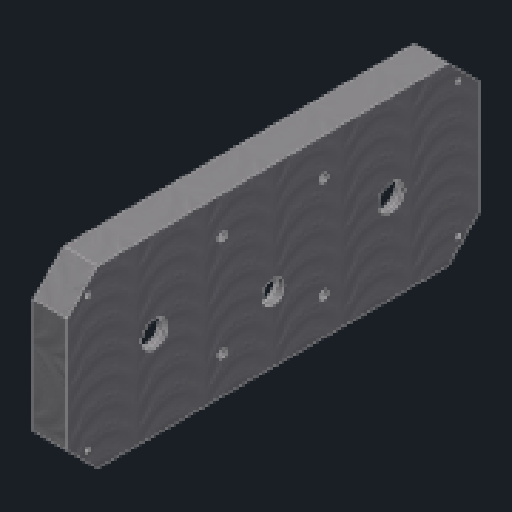
# Autodesk Inventor part: CAJA
Saved by Autodesk Inventor 2024.3 (Build 283343000, 343)
## iProperties
Created: 2024-06-29
Part Number: CAJA
Material: Steel, Mild, Welded
Document SubType Name: Modeling
Designer: Niler
Density: 7.85 g/cm^3
Appearance: Weld - Steel Mild
Author: Niler
Autodesk Inventor part; units mm, degrees
ref_plane "YZ Plane" through (0, 0, 0) normal (1, 0, 0) x (0, 1, 0)
ref_plane "XZ Plane" through (0, 0, 0) normal (0, 1, 0) x (-1, 0, 0)
ref_plane "XY Plane" through (0, 0, 0) normal (0, 0, 1) x (1, 0, 0)
sketch "Sketch1" plane through (0, 0, 0) normal (1, 0, 0) x (0, 1, 0)
  line L0 (-57.5, 135) -> (57.5, 135)
  line L1 (57.5, 135) -> (57.5, -135)
  line L2 (57.5, -135) -> (-57.5, -135)
  line L3 (-57.5, -135) -> (-57.5, 135)
  line L4 (-57.5, 135) -> (57.5, -135) construction
  line L5 (57.5, 135) -> (-57.5, -135) construction
  circle A0 centre (0, 77.5) radius 3.925
  circle A1 centre (0, -77.5) radius 3.925
  circle A2 centre (-15, 0) radius 5
  line L6 (0, 77.5) -> (0, -77.5) construction
  line L7 (51.5, -129) -> (51.5, 129)
  line L8 (51.5, 129) -> (-51.5, 129)
  line L9 (-51.5, 129) -> (-51.5, -129)
  line L10 (-51.5, -129) -> (51.5, -129)
  point P0 (0, 0)
  dimension "d0" = 155
  dimension "d1" = 7.85
  dimension "d2" = 270
  dimension "d3" = 115
  dimension "d4" = 6
  dimension "d35" = 10
  dimension "d36" = 15
  constraints: 22 end point, 4 parallel, 3 centre point, 3 midpoint, 2 perpendicular, 1 equal radius, 1 horizontal, 1 horizontal alignment, 1 vertical, 1 vertical alignment, 3 other
  measures "d0" distance of L6.end L6.start
  measures "d1" diameter of A0
  measures "d2" distance between parallel lines of L2 L0
  measures "d3" distance of L0.start L0.end
  measures "d4" distance between parallel lines of L1 L7
  measures "d35" diameter of A2
  measures "d36" distance of A2.centre point (0, 0)
extrude "Extrusion1" add sketch "Sketch1" along normal blind 8 contours L0 L1 L2 L3 | A0 | A1 | L10 L9 L8 L7
extrude "Extrusion2" add sketch "Sketch1" against normal blind 14.4 contours L0 L1 L2 L3
sketch "Sketch2" plane through (8, 0, 0) normal (1, 0, 0) x (0, 0, -1)
  line L0 (135, -57.5) -> (135, 57.5) projected
  line L1 (135, 57.5) -> (-135, 57.5) projected
  line L2 (-135, 57.5) -> (-135, -57.5) projected
  line L3 (-135, -57.5) -> (135, -57.5) projected
  line L4 (-33.234, -33.234) -> (33.234, -33.234) construction
  line L5 (33.234, -33.234) -> (33.234, 33.234) construction
  line L6 (33.234, 33.234) -> (-33.234, 33.234) construction
  line L7 (-33.234, 33.234) -> (-33.234, -33.234) construction
  line L8 (-33.234, -33.234) -> (33.234, 33.234) construction
  line L9 (33.234, -33.234) -> (-33.234, 33.234) construction
  circle A0 centre (0, 0) radius 47 construction
  circle A1 centre (33.234, 33.234) radius 2.75
  circle A2 centre (-33.234, 33.234) radius 2.75
  circle A3 centre (0, 0) radius 47 construction
  circle A4 centre (-33.234, -33.234) radius 2.75
  circle A5 centre (0, 0) radius 47 construction
  circle A6 centre (33.234, -33.234) radius 2.75
  circle A7 centre (0, 0) radius 47 construction
  point P0 (0, 0)
  point P1 (0, 0)
  dimension "d12" = 94
  dimension "d13" = 5.5
  dimension "d16" = 360
  constraints: 12 end point, 7 coincident, 4 centre point, 2 parallel, 2 perpendicular, 1 horizontal, 1 midpoint, 31 other
  measures "d13" diameter of A1
extrude "Extrusion3" cut sketch "Sketch2" against normal through all contours A1 | A2 | A4 | A6
sketch "Sketch3" plane through (0, 0, 0) normal (-1, 0, 0) x (0, 0, 1)
  circle A0 centre (33.234, -33.234) radius 2.75 projected
  circle A1 centre (33.234, 33.234) radius 2.75 projected
  circle A2 centre (-33.234, -33.234) radius 2.75 projected
  circle A3 centre (-33.234, 33.234) radius 2.75 projected
  line L0 (-129, -51.5) -> (129, -51.5) projected
  line L1 (129, -51.5) -> (129, 51.5) projected
  line L2 (129, 51.5) -> (-129, 51.5) projected
  line L3 (-129, 51.5) -> (-129, -51.5) projected
  circle A4 centre (0, -15) radius 5 projected
  circle A5 centre (-33.234, 33.234) radius 4.5
  circle A6 centre (33.234, 33.234) radius 2.75 projected
  circle A7 centre (33.234, 33.234) radius 4.5
  circle A8 centre (-33.234, -33.234) radius 4.5
  circle A9 centre (33.234, -33.234) radius 4.5
  point P0 (0, 0)
  dimension "d20" = 9
  constraints: 4 centre point, 4 coincident, 3 equal radius
  measures "d20" diameter of A5
extrude "Extrusion4" cut sketch "Sketch3" against normal blind 3 contours A0 | A1 | A2 | A3 | A5 | A7 | A8 | A9
sketch "Sketch4" plane through (8, 0, 0) normal (1, 0, 0) x (0, 0, -1)
  circle A0 centre (-33.234, -33.234) radius 2.75 projected
  circle A1 centre (-33.234, 33.234) radius 2.75 projected
  circle A2 centre (33.234, -33.234) radius 2.75 projected
  circle A3 centre (33.234, 33.234) radius 2.75 projected
  line L0 (135, -57.5) -> (135, 57.5) projected
  line L1 (135, 57.5) -> (-135, 57.5) projected
  line L2 (-135, 57.5) -> (-135, -57.5) projected
  line L3 (-135, -57.5) -> (135, -57.5) projected
  circle A4 centre (0, -15) radius 5 projected
  circle A5 centre (0, -15) radius 7.5
  point P0 (0, 0)
  dimension "d24" = 15
  constraints: 1 centre point, 1 coincident
  measures "d24" diameter of A5
extrude "Extrusion5" cut sketch "Sketch4" against normal through all contours A4 | A5
chamfer "Chamfer2" distance 25 angle 45 8 edges at (-7.2, 51.5, -129) (-7.2, -51.5, -129) (-7.2, -51.5, 129) (-7.2, 51.5, 129) (-3.2, 57.5, -135) (-3.2, -57.5, -135) (-3.2, -57.5, 135) (-3.2, 57.5, 135)
sketch "Sketch6" plane through (-14.4, 0, 0) normal (-1, 0, 0) x (0, 0, 1)
  line L0 (110, 57.5) -> (135, 32.5) projected
  line L1 (110, 57.5) -> (-110, 57.5) projected
  line L2 (-135, 32.5) -> (-110, 57.5) projected
  line L3 (-135, 32.5) -> (-135, -32.5) projected
  line L4 (-110, -57.5) -> (-135, -32.5) projected
  line L5 (-110, -57.5) -> (110, -57.5) projected
  line L6 (135, -32.5) -> (110, -57.5) projected
  line L7 (135, -32.5) -> (135, 32.5) projected
  line L8 (-129, -26.5) -> (-129, 26.5) projected
  line L9 (-104, 51.5) -> (-129, 26.5) projected
  line L10 (-104, 51.5) -> (104, 51.5) projected
  line L11 (129, 26.5) -> (104, 51.5) projected
  line L12 (129, 26.5) -> (129, -26.5) projected
  line L13 (104, -51.5) -> (129, -26.5) projected
  line L14 (104, -51.5) -> (-104, -51.5) projected
  line L15 (-129, -26.5) -> (-104, -51.5) projected
  line L16 (119.5, -42) -> (-119.5, -42)
  line L17 (-119.5, -42) -> (-119.5, 42)
  line L18 (-119.5, 42) -> (119.5, 42)
  line L19 (119.5, 42) -> (119.5, -42)
  circle A0 centre (0, 0) radius 10.3
  line L20 (119.5, -42) -> (-119.5, 42) construction
  line L21 (-119.5, -42) -> (119.5, 42) construction
  circle A1 centre (-119.5, 42) radius 1.5
  circle A2 centre (-119.5, -42) radius 1.5
  circle A3 centre (119.5, -42) radius 1.5
  circle A4 centre (119.5, 42) radius 1.5
  line L22 (-122.5, 45) -> (-116.5, 39)
  dimension "d32" = 3
  constraints: 14 end point, 5 centre point, 5 coincident, 5 midpoint, 3 equal radius, 2 parallel, 1 horizontal, 1 perpendicular
  measures "d32" diameter of A1
extrude "Extrusion7" cut sketch "Sketch6" against normal through all contours A2 L16 L17 | L17 L16 A2 | A1 L22 L17 | L17 L22 A1 | L22 L18 A1 | L22 A1 L18 | A3 L19 L16 | L16 L19 A3 | A4 L19 L18 | L18 L19 A4
sketch "Sketch12" plane through (0, 0, 0) normal (-1, 0, 0) x (0, 0, 1)
  circle A0 centre (-77.5, 0) radius 3.925 projected
  circle A1 centre (77.5, 0) radius 3.925 projected
  circle A2 centre (-77.5, 0) radius 11.15
  circle A3 centre (77.5, 0) radius 11.15
  point P0 (0, 0)
  dimension "d61" = 22.3
  constraints: 2 centre point, 2 coincident, 1 equal radius
  measures "d61" diameter of A2
extrude "Extrusion13" cut sketch "Sketch12" against normal blind 5 contours A0 | A1 | A2 | A3
sketch "Sketch13" plane through (5, 0, -77.5) normal (-1, 0, 0) x (0, 0, 1)
  circle A0 centre (0, 0) radius 11.15 projected
  circle A1 centre (155, 0) radius 11.15 projected
  circle A2 centre (0, 0) radius 8.5
  circle A3 centre (155, 0) radius 8.5
  point P0 (77.5, 0)
  dimension "d64" = 17
  dimension "d65" = 17
  constraints: 2 centre point, 2 coincident
  measures "d64" diameter of A2
  measures "d65" diameter of A3
extrude "Extrusion14" cut sketch "Sketch13" against normal through all contours A2 | A3
sketch "Sketch14" plane through (0, 0, 0) normal (-1, 0, 0) x (0, 0, 1)
  circle A0 centre (0, -15) radius 7.5 projected
  circle A1 centre (0, -15) radius 9.65
  point P0 (0, 0)
  dimension "d68" = 19.3
  constraints: 1 centre point, 1 coincident
  measures "d68" diameter of A1
extrude "Extrusion15" cut sketch "Sketch14" against normal blind 3
ref_plane "Work Plane1" through (-8.4, 0, 0) normal (-1, 0, 0) x (0, 0, 1)
sketch "Sketch15" plane through (-8.4, 0, 0) normal (-1, 0, 0) x (0, 0, 1)
  circle A0 centre (-119.5, 42) radius 1.5 projected
  line L0 (-120.3667, 45.2345) -> (-117.1322, 44.3678)
  line L1 (-117.1322, 44.3678) -> (-116.2655, 41.1333)
  line L2 (-116.2655, 41.1333) -> (-118.6333, 38.7655)
  line L3 (-118.6333, 38.7655) -> (-121.8678, 39.6322)
  line L4 (-121.8678, 39.6322) -> (-122.7345, 42.8667)
  line L5 (-122.7345, 42.8667) -> (-120.3667, 45.2345)
  line L6 (-135, 32.5) -> (-110, 57.5) projected
  line L7 (-117.1322, 44.3678) -> (-120.1322, 47.3678)
  line L8 (-121.8678, 39.6322) -> (-124.8678, 42.6322)
  point P0 (0, 0)
  dimension "d72" = 5.8
  constraints: 16 end point, 2 perpendicular, 2 point on line, 1 coincident, 1 parallel, 13 other
  measures "d72" distance between parallel lines of L2 L5
extrude "Extrusion16" cut sketch "Sketch15" along normal blind 3
mirror "Mirror1" about plane through (0, 0, 0) normal (0, 1, 0) of "Extrusion16"
mirror "Mirror2" about plane through (0, 0, 0) normal (0, 0, 1) of "Extrusion16", "Mirror1"
sketch "Sketch16" plane through (0, 0, 0) normal (-1, 0, 0) x (0, 0, 1)
  circle A0 centre (-21.0923, 23.1558) radius 4
  circle A1 centre (-37.6476, -46.4615) radius 4
  circle A2 centre (0, -15) radius 9.65 projected
  circle A3 centre (77.5, 0) radius 11.15 projected
  circle A4 centre (-77.5, 0) radius 11.15 projected
  line L0 (129, 26.5) -> (104, 51.5) projected
  line L1 (104, 51.5) -> (-104, 51.5) projected
  line L2 (-104, 51.5) -> (-129, 26.5) projected
  line L3 (-129, 26.5) -> (-129, -26.5) projected
  line L4 (-129, -26.5) -> (-104, -51.5) projected
  line L5 (-104, -51.5) -> (104, -51.5) projected
  line L6 (104, -51.5) -> (129, -26.5) projected
  line L7 (129, -26.5) -> (129, 26.5) projected
  circle A5 centre (-33.234, -33.234) radius 4.5 projected
  circle A6 centre (33.234, 33.234) radius 4.5 projected
  circle A7 centre (33.234, -33.234) radius 4.5 projected
  circle A8 centre (-33.234, 33.234) radius 4.5 projected
  line L8 (0, 0) -> (0, 21.7983)
  circle A9 centre (21.0923, 23.1558) radius 4
  circle A10 centre (37.6476, -46.4615) radius 4
  dimension "d75" = 8
  dimension "d76" = 8
  constraints: 4 centre point, 2 end point, 2 symmetric about line, 1 vertical, 2 other
  measures "d75" diameter of A0
  measures "d76" diameter of A1
extrude "Extrusion17" add sketch "Sketch16" along normal up to surface (14.4 mm away) contours A0 | A1 | A9 | A10
sketch "Sketch17" plane through (-14.4, 23.1558, -21.0923) normal (-1, 0, 0) x (0, 0, 1)
  circle A0 centre (0, 0) radius 4 projected
  circle A1 centre (42.1847, 0) radius 4 projected
  circle A2 centre (-16.5553, -69.6173) radius 4 projected
  circle A3 centre (58.7399, -69.6173) radius 4 projected
  circle A4 centre (-16.5553, -69.6173) radius 1.5
  circle A5 centre (58.7399, -69.6173) radius 1.5
  circle A6 centre (0, 0) radius 1.5
  circle A7 centre (42.1847, 0) radius 1.5
  point P0 (21.0923, -23.1558)
  dimension "d79" = 3
  constraints: 4 centre point, 4 coincident, 3 equal radius
  measures "d79" diameter of A6
extrude "Extrusion18" cut sketch "Sketch17" against normal through all contours A4 | A5 | A6 | A7
chamfer "Chamfer3" distance 3 angle 75 4 edges at (0, -46.4615, -41.6476) (0, 23.1558, -25.0923) (0, 23.1558, 17.0923) (0, -46.4615, 33.6476) measured on face at (0, 23.1558, 16.5923) measured on face at (0, -46.4615, 33.1476) measured on face at (0, 23.1558, -25.5923) measured on face at (0, -46.4615, -42.1476)
body "Solid1"
